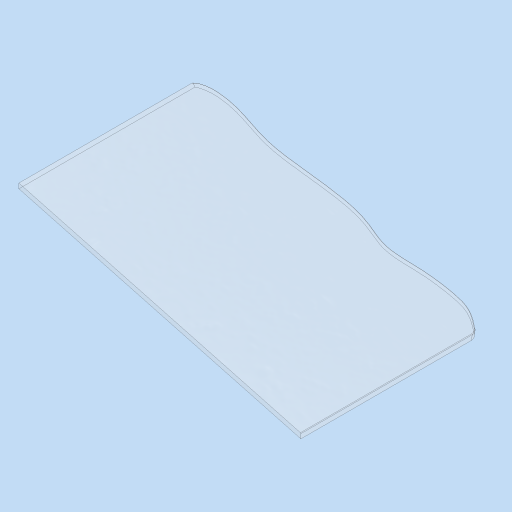
# Autodesk Inventor part: 유리
Saved by Autodesk Inventor 2024 (Build 280153000, 153)
## iProperties
Created: 2024-01-19
Part Number: 유리
Material: 아크릴
Document SubType Name: Modeling
Designer: KBU
Density: 1.188 g/cm^3
Appearance: 투명 - 선명
Author: KBU
Autodesk Inventor part; units mm, degrees
ref_plane "YZ Plane" through (0, 0, 0) normal (1, 0, 0) x (0, 1, 0)
ref_plane "XZ Plane" through (0, 0, 0) normal (0, 1, 0) x (-1, 0, 0)
ref_plane "XY Plane" through (0, 0, 0) normal (0, 0, 1) x (1, 0, 0)
sketch "스케치1" plane through (0, 0, 0) normal (0, 0, 1) x (1, 0, 0)
  line L0 (0, 0) -> (0, 1.5)
  line L1 (0, 1.5) -> (-85, 24.2757)
  line L2 (-85, 24.2757) -> (-85, 22.7757)
  line L3 (-85, 22.7757) -> (0, 0)
  line L4 (-4.5515, 0) -> (6.2114, 0)
  point P0 (0, 0.75)
  point P1 (-85, 23.5257)
  dimension "d0" = 15
  dimension "d1" = 1.5
  dimension "d2" = 85
  constraints: 10 end point, 2 midpoint, 2 parallel, 1 horizontal, 1 point on line, 1 vertical
  measures "d0" angle of L3 L4
  measures "d1" distance of L1.end L2.end
  measures "d2" horizontal distance of point (0, 0.75) point (-85, 23.526)
extrude "돌출1" add sketch "스케치1" against normal blind 105
sketch "스케치2" plane through (0, 1.5, 0) normal (0.2588, 0.9659, 0) x (0.9659, -0.2588, 0)
  line L0 (-87.9985, 0) -> (-87.9985, 105) projected
  line L1 (0.3882, 0) -> (0.3882, 105) projected
  spline S0 degree 4 poles (-87.9985, 52.5) (-86.205, 55.4067) (-76.8714, 56.646) (-70.0535, 53.3359) (-57.0807, 54.7242) (-36.5304, 57.94) (-31.1569, 52.3064) (-20.5582, 56.3272) (-11.3877, 56.8091) (-5.5108, 57.1936) (-2.2705, 54.3001) (0.3882, 52.5) knots 0 0 0 0 0 0.235936 0.353495 0.472108 0.596349 0.719338 0.802737 0.888043 1 1 1 1 1
  line L2 (-9.2686, 59.038) -> (10.045, 45.962) construction
  arc A0 (-6.5887, 58.4361) -> (8.4909, 48.2267) centre (23.8158, 87.1033) ccw construction
  line L3 (-16.7235, 57.4254) -> (-0.3146, 56.0774) construction
  arc A1 (-2.5664, 55.0363) -> (-14.6718, 56.0308) centre (-9.8047, 41.1019) ccw construction
  line L4 (-87.9985, 52.5) -> (-129.1684, 51.5107)
  line L5 (-129.1684, 51.5107) -> (-110.0739, 114.0314)
  line L6 (-110.0739, 114.0314) -> (85.9028, 105)
  line L7 (85.9028, 105) -> (0.3882, 52.5)
  point P0 (-83.0539, 55.1625)
  point P1 (-75.1656, 55.3033)
  point P2 (-68.1749, 54.3668)
  point P3 (-57.3109, 54.8527)
  point P4 (-37.54, 55.8207)
  point P5 (-29.1151, 54.2549)
  point P6 (-18.466, 56.1281)
  point P7 (-8.519, 56.7514)
  constraints: 12 end point, 6 midpoint, 2 centre point, 2 point on circle, 14 other
extrude "돌출2" cut sketch "스케치2" against normal blind 105
fillet "모깎기1" radius 2 1 edges at (0, 0.7501, -52.6322)
fillet "모깎기2" radius 0.2 3 edges at (-42.8374, 12.9782, -56.1807) (-0.2384, 1.5639, -52.6527) (0, 1.5, -25.8391)
